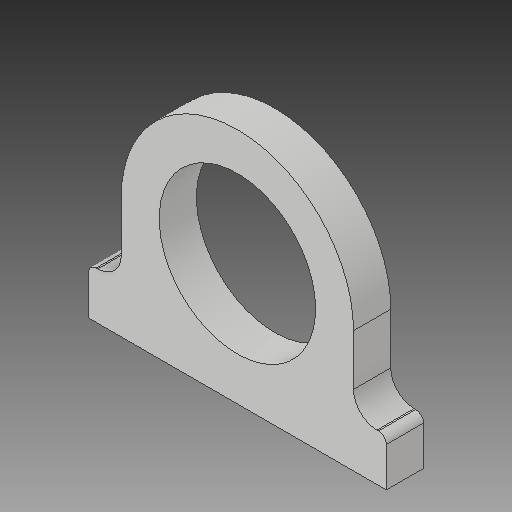
# Autodesk Inventor part: SuporteAquecedor
Saved by Autodesk Inventor 2018 (Build 220112000, 112)
## iProperties
Created: 2018-07-23
Part Number: SuporteAquecedor
Material: Genérico
Document SubType Name: Modeling
Designer: Usuario
Density: 1 g/cm^3
Appearance: Padrão
Mass: 20.8536 g
Surface Area: 78.7699 cm^2
Volume: 20.8536 cm^3
Author: Usuario
Autodesk Inventor part; units mm, degrees
ref_plane "YZ Plane" through (0, 0, 0) normal (1, 0, 0) x (0, 1, 0)
ref_plane "XZ Plane" through (0, 0, 0) normal (0, 1, 0) x (-1, 0, 0)
ref_plane "XY Plane" through (0, 0, 0) normal (0, 0, 1) x (1, 0, 0)
sketch "Esboço1" plane through (0, 0, 0) normal (0, 0, 1) x (1, 0, 0)
  circle A0 centre (-38.1, 31.06) radius 20
  line L0 (0, 0) -> (-76.2, 0)
  line L1 (-76.2, 0) -> (-76.2, 10.06)
  line L2 (0, 10.06) -> (0, 0)
  line L3 (-67.8019, 31.06) -> (-67.8019, 18.06)
  line L4 (-73.8019, 12.06) -> (-74.2, 12.06)
  line L5 (-38.1, 31.06) -> (-38.1, 69.4072) construction
  line L6 (-8.3981, 31.06) -> (-8.3981, 18.06)
  line L7 (-2.3981, 12.06) -> (-2, 12.06)
  arc A1 (-8.3981, 31.06) -> (-67.8019, 31.06) centre (-38.1, 31.06) ccw
  arc A2 (-73.8019, 12.06) -> (-67.8019, 18.06) centre (-73.8019, 18.06) ccw
  arc A3 (-8.3981, 18.06) -> (-2.3981, 12.06) centre (-2.3981, 18.06) ccw
  arc A4 (0, 10.06) -> (-2, 12.06) centre (-2, 10.06) ccw
  arc A5 (-74.2, 12.06) -> (-76.2, 10.06) centre (-74.2, 10.06) ccw
  point P0 (-67.8019, 12.06)
  point P1 (-8.3981, 12.06)
  point P2 (0, 12.06)
  point P3 (-76.2, 12.06)
  dimension "d4" = 40
  dimension "d8" = 31.06
  dimension "d9" = 6
  dimension "d10" = 76.2
  dimension "d11" = 2
  constraints: 16 end point, 10 point on circle, 9 tangent, 8 point on line, 6 centre point, 2 equal radius, 2 perpendicular, 2 symmetric about line, 2 vertical, 1 horizontal, 1 parallel
  measures "d4" diameter of A0
  measures "d8" distance from line of L0 L5.start
  measures "d9" radius of A2
  measures "d10" distance of L0.start L0.end
  measures "d11" radius of A4
extrude "Extrusão1" add sketch "Esboço1" against normal blind 9.52
